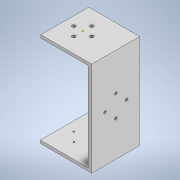
# Autodesk Inventor part: sidebracket
Saved by Autodesk Inventor 2022.2 (Build 262287030, 287C)
## iProperties
Created: 2022-03-11
Part Number: sidebracket
Material: Generic
Document SubType Name: Modeling
Designer: Tapendra
Density: 1 g/cm^3
Appearance: Default
Author: Tapendra
Autodesk Inventor part; units mm, degrees
ref_plane "YZ Plane" through (0, 0, 0) normal (1, 0, 0) x (0, 1, 0)
ref_plane "XZ Plane" through (0, 0, 0) normal (0, 1, 0) x (-1, 0, 0)
ref_plane "XY Plane" through (0, 0, 0) normal (0, 0, 1) x (1, 0, 0)
sketch "Sketch1" plane through (0, 0, 0) normal (0, 0, 1) x (1, 0, 0)
  line L0 (19.808, 75.5) -> (19.808, -72.5)
  line L1 (19.808, 75.5) -> (167.808, 75.5) construction
  line L2 (19.808, -72.5) -> (-60.192, -72.5)
  line L3 (-60.192, -72.5) -> (-60.192, -77.5)
  line L4 (-60.192, -72.5) -> (-55.192, -72.5) construction
  line L5 (-60.192, -77.5) -> (25.808, -77.5)
  line L6 (25.808, -77.5) -> (25.808, 80.5)
  line L7 (25.808, 80.5) -> (-59.192, 80.5)
  line L8 (-59.192, 80.5) -> (-59.192, 75.5)
  line L9 (-59.192, 75.5) -> (19.808, 75.5)
  point P0 (0, 0)
  dimension "d0" = 148
  dimension "d1" = 90
  dimension "d2" = 80
  dimension "d3" = 90
  dimension "d4" = 5
  dimension "d5" = 90
  dimension "d6" = 86
  dimension "d7" = 90
  dimension "d8" = 158
  dimension "d9" = 90
  dimension "d10" = 85
  dimension "d11" = 90
  dimension "d12" = 5
  dimension "d13" = 90
  dimension "d45" = 72.5
  constraints: 20 end point, 7 perpendicular, 2 horizontal, 2 vertical
  measures "d0" distance of L0.start L0.end
  measures "d1" angle of L0 L1
  measures "d2" distance of L0.end L2.end
  measures "d3" angle of L0 L2
  measures "d4" distance of L2.end L3.end
  measures "d5" angle of L3 L4
  measures "d6" distance of L3.end L5.end
  measures "d7" angle of L5 L3
  measures "d8" distance of L5.end L6.end
  measures "d9" angle of L6 L5
  measures "d10" distance of L6.end L7.end
  measures "d11" angle of L7 L6
  measures "d12" distance of L7.end L8.end
  measures "d13" angle of L8 L7
  measures "d45" distance from line of L2 point (0, 0)
extrude "Extrusion1" add sketch "Sketch1" along normal mid plane 80
sketch "Sketch3" plane through (-59.192, 80.5, 40) normal (0, 1, 0) x (1, 0, 0)
  line L0 (60, 80) -> (0, 80)
  line L1 (30, 80) -> (30, 0) construction
  line L2 (60, 0) -> (0, 0)
  line L3 (30, 80) -> (120, 80) construction
  line L4 (85, 80) -> (85, 0) projected
  line L5 (85, 0) -> (0, 0) projected
  line L6 (0, 80) -> (85, 80) projected
  point P0 (59.817, 40)
  point P1 (15, 40)
  point P2 (30, 40)
  point P3 (30, 25)
  point P4 (45, 40)
  point P5 (30, 55)
  dimension "d30" = 90
  dimension "d31" = 55
  dimension "d32" = 40
  dimension "d33" = 15
  dimension "d36" = 360
  constraints: 8 end point, 3 midpoint, 2 point on line, 1 horizontal, 5 other
  measures "d30" angle of L1 L3
  measures "d31" distance between parallel lines of L4 L1
  measures "d32" distance from line of L2 point (15, 40)
  measures "d33" distance from line of point (15, 40) L1
hole "Hole2" at (-14.192, 80.5, 0) at (-29.192, 80.5, 15) at (-44.192, 80.5, 0) at (-29.192, 80.5, -15) direction (0, -1, 0) diameter 2.459 depth 5 counterbore diameter 6 counterbore depth 1 thread size "M3x0.5" class "6H" standard "ANSI Metric M Profile"
sketch "Sketch5" plane through (-60.192, -77.5, 40) normal (0, -1, 0) x (1, 0, 0)
  line L0 (31, -80) -> (31, 0) construction
  line L1 (31, -80) -> (111, -80) construction
  line L2 (86, -80) -> (86, 0) projected
  line L3 (0, 0) -> (86, 0) projected
  line L4 (86, -80) -> (0, -80) projected
  point P0 (60.192, -40)
  point P1 (31, -40)
  point P2 (16, -40)
  point P3 (31, -55)
  point P4 (46, -40)
  point P5 (31, -25)
  dimension "d48" = 90
  dimension "d49" = 55
  dimension "d50" = 15
  dimension "d53" = 360
  constraints: 4 end point, 2 point on line, 1 horizontal, 1 horizontal alignment, 1 midpoint, 1 perpendicular, 5 other
  measures "d48" angle of L1 L0
  measures "d49" distance from line of L2 point (31, -40)
  measures "d50" distance of point (16, -40) point (31, -40)
hole "Hole3" at (-29.192, -77.5, 15) at (-29.192, -77.5, -15) at (-44.192, -77.5, 0) at (-14.192, -77.5, 0) direction (0, 1, 0) diameter 2.459 depth 5 counterbore diameter 6 counterbore depth 1 thread size "M3x0.5" class "6H" standard "ANSI Metric M Profile"
sketch "Sketch6" plane through (19.808, -72.5, 40) normal (-1, 0, 0) x (0, 0, 1)
  point P0 (-40, 72.5)
  point P1 (-40, 90.53)
  point P2 (-58.03, 72.5)
  point P3 (-40, 54.47)
  point P4 (-21.97, 72.5)
  dimension "d62" = 18.03
  dimension "d65" = 360
  constraints: 1 vertical alignment, 5 other
  measures "d62" distance of point (-40, 90.53) point (-40, 72.5)
hole "Hole4" at (19.808, 0, -18.03) at (19.808, -18.03, 0) at (19.808, 0, 18.03) at (19.808, 18.03, 0) direction (1, 0, 0) diameter 4.134 end through all counterbore diameter 9.93 counterbore depth 3 thread size "M5x0.8" class "6H" standard "ANSI Metric M Profile"
body "Solid1"
